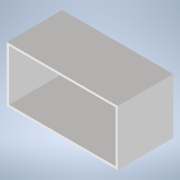
# Autodesk Inventor part: bottom
Saved by Autodesk Inventor 2021 (Build 250183000, 183)
## iProperties
Created: 2021-03-15
Part Number: bottom
Material: Všeobecné
Document SubType Name: Modeling
Designer: kanyk
Density: 1 g/cm^3
Appearance: Výchozí
Author: kanyk
Autodesk Inventor part; units mm, degrees
ref_plane "YZ Plane" through (0, 0, 0) normal (1, 0, 0) x (0, 1, 0)
ref_plane "XZ Plane" through (0, 0, 0) normal (0, 1, 0) x (-1, 0, 0)
ref_plane "XY Plane" through (0, 0, 0) normal (0, 0, 1) x (1, 0, 0)
sketch "Náčrt1" plane through (0, 0, 0) normal (0, 0, 1) x (1, 0, 0)
  line L0 (0, 0) -> (100, 0)
  line L1 (100, 0) -> (100, 50)
  line L2 (100, 50) -> (0, 50)
  line L3 (0, 50) -> (0, 0)
  dimension "d0" = 100
  dimension "d1" = 50
  constraints: 8 end point, 2 parallel, 1 horizontal, 1 perpendicular
  measures "d0" distance of L2.end L1.end
  measures "d1" distance of L1.end L0.end
extrude "Vysunutí1" add sketch "Náčrt1" along normal blind 49
sketch "Náčrt2" plane through (0, 0, 49) normal (0, 0, 1) x (1, 0, 0)
  line L0 (2, 2) -> (98, 2)
  line L1 (98, 2) -> (98, 48)
  line L2 (98, 48) -> (2, 48)
  line L3 (2, 48) -> (2, 2)
  point P0 (0, 0)
  dimension "d4" = 96
  dimension "d5" = 46
  constraints: 8 end point, 2 parallel, 1 horizontal, 1 perpendicular
  measures "d4" distance of L2.end L1.end
  measures "d5" distance of L1.end L0.end
extrude "Vysunutí2" cut sketch "Náčrt2" against normal blind 48
